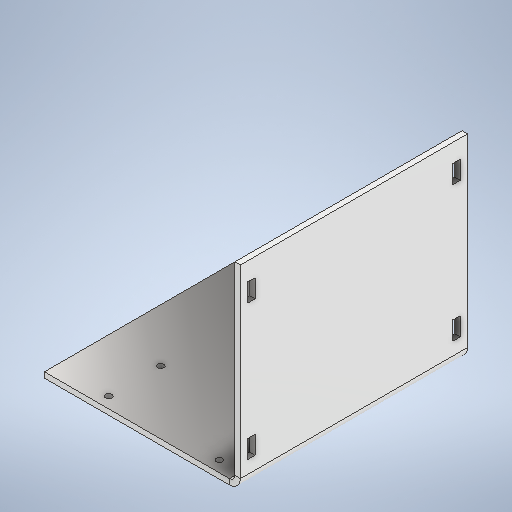
# Autodesk Inventor part: Face with CWT hole
Saved by Autodesk Inventor 2025 (Build 290162000, 162)
## iProperties
Created: 2025-08-10
Part Number: Face with CWT hole
Material: Steel, Carbon
Document SubType Name: Sheet Metal
Designer: yshis
Density: 7.85 g/cm^3
Sheet Metal Rule: Default
Appearance: Semi-Polished
Author: yshis
Autodesk Inventor part; units mm, degrees
ref_plane "YZ Plane" through (0, 0, 0) normal (1, 0, 0) x (0, 1, 0)
ref_plane "XZ Plane" through (0, 0, 0) normal (0, 1, 0) x (-1, 0, 0)
ref_plane "XY Plane" through (0, 0, 0) normal (0, 0, 1) x (1, 0, 0)
sketch "Sketch1" plane through (0, 0, 0) normal (0, 1, 0) x (-1, 0, 0)
  line L0 (0, 0) -> (107, 0)
  line L1 (107, 0) -> (107, -124)
  line L2 (107, -124) -> (0, -124)
  line L3 (0, -124) -> (0, 0)
  point P0 (53.5, -124)
  dimension "d0" = 107
  dimension "d1" = 124
  measures "d0" distance of L1.end L2.end
  measures "d1" distance of L0.end L1.end
extrude "Plate1" add sketch "Sketch1" along normal blind 3
sketch "Sketch2" plane through (-3, 0, -124) normal (1, 0, 0) x (0, 1, 0)
  line L0 (0, 124) -> (0, 0)
  line L1 (0, 0) -> (107, 0)
  line L2 (107, 0) -> (107, 124)
  line L3 (107, 124) -> (0, 124)
  constraints: 6 end point, 1 horizontal, 1 perpendicular, 1 vertical
edge flange "Flange1" height 107 angle 90 thickness 3 bend radius 3 thickness toward (1, 0, 0) relief tear relief width 3 relief depth 1.5 edges at (0, 3, -62) wall of the first edge with corners at (-3, 0, 0) (-3, 0, -124) (-3, 107, -124) (-3, 107, 0)
bend "Bend1"
corner "Corner1"
sketch "Sketch6" plane through (0, 0, 0) normal (0, -1, 0) x (1, 0, 0)
  circle A0 centre (-78, -118) radius 1.75
  line L0 (-107, -124) -> (-107, 0) projected
  line L1 (-6, -124) -> (-107, -124) projected
  circle A1 centre (-78, -34.5) radius 1.75
  circle A2 centre (-17.5, -118) radius 1.75
  circle A3 centre (-17.5, -34.5) radius 1.75
  circle A4 centre (-78, -6) radius 1.75
  line L2 (-107, 0) -> (-6, 0) projected
  circle A5 centre (-78, -89.5) radius 1.75
  circle A6 centre (-17.5, -6) radius 1.75
  circle A7 centre (-17.5, -89.5) radius 1.75
  point P0 (0, 0)
  dimension "d79" = 3.5
  dimension "d80" = 29
  dimension "d81" = 6
  dimension "d84" = 83.5
  dimension "d87" = 60.5
  dimension "d113" = 3.5
  dimension "d114" = 6
  dimension "d115" = 29
  dimension "d118" = 83.5
  dimension "d121" = 60.5
  constraints: 8 centre point, 2 horizontal, 2 vertical, 12 other
  measures "d79" diameter of A0
  measures "d80" distance from line of L0 A0.centre
  measures "d81" distance from line of L1 A0.centre
  measures "d84" distance of A0.centre A1.centre
  measures "d87" distance of A0.centre A2.centre
  measures "d113" diameter of A4
  measures "d114" distance from line of L2 A4.centre
  measures "d115" distance from line of L0 A4.centre
  measures "d118" distance of A4.centre A5.centre
  measures "d121" distance of A4.centre A6.centre
extrude "Cut4" cut sketch "Sketch6" against normal blind 3
sketch "Sketch7" plane through (0, 107, 0) normal (1, 0, 0) x (0, 0, -1)
  line L0 (120, -84) -> (116, -84)
  line L1 (116, -84) -> (116, -94)
  line L2 (116, -94) -> (120, -94)
  line L3 (120, -94) -> (120, -84)
  line L4 (124, 0) -> (124, -101) projected
  line L5 (124, -107) -> (0, -107) projected
  line L6 (120, -10) -> (116, -10)
  line L7 (116, -10) -> (116, -20)
  line L8 (116, -20) -> (120, -20)
  line L9 (120, -20) -> (120, -10)
  line L10 (8, -84) -> (4, -84)
  line L11 (4, -84) -> (4, -94)
  line L12 (4, -94) -> (8, -94)
  line L13 (8, -94) -> (8, -84)
  line L14 (8, -10) -> (4, -10)
  line L15 (4, -10) -> (4, -20)
  line L16 (4, -20) -> (8, -20)
  line L17 (8, -20) -> (8, -10)
  point P0 (124, -27)
  point P1 (124, -33)
  point P2 (12, -101)
  point P3 (12, -107)
  point P4 (12, -27)
  point P5 (12, -33)
  dimension "d92" = 10
  dimension "d93" = 4
  dimension "d94" = 4
  dimension "d95" = 13
  dimension "d105" = 74
  dimension "d108" = 112
  constraints: 32 end point, 2 horizontal, 2 parallel, 1 perpendicular, 1 vertical, 30 other
  measures "d92" distance of L0.end L1.end
  measures "d93" distance of L0.start L0.end
  measures "d94" distance between parallel lines of L4 L3
  measures "d95" distance between parallel lines of L5 L2
  measures "d105" distance of L0.start L6.start
  measures "d108" distance of L0.start L10.start
extrude "Extrusion1" cut sketch "Sketch7" against normal blind 3
equation "\"d114\" = d81"
equation "\"d115\" = d80"
equation "\"d118\" = d84"
equation "\"d121\" = d87"
equation "\"d90\" = Thickness"
equation "\"d108\" = d1 - d93 - 2 * d94"
equation "\"d24\" = Thickness"
equation "\"d25\" = BendReliefWidth"
equation "\"d26\" = BendReliefDepth"
equation "\"d27\" = MinimumRemnant"
equation "\"d28\" = TransitionRadius"
equation "\"d29\" = d0"
equation "\"d31\" = BendRadius"
equation "\"d32\" = CornerReliefSize"
equation "\"d33\" = GapSize"
equation "\"d34\" = JacobiRadiusSize"
equation "\"BendRadius\" = Thickness"
equation "\"BendReliefWidth\" = Thickness"
equation "\"BendReliefDepth\" = 0.5 * Thickness"
equation "\"CornerReliefSize\" = 4 * Thickness"
equation "\"MinimumRemnant\" = 2 * Thickness"
equation "\"TransitionRadius\" = BendRadius"
equation "\"JacobiRadiusSize\" = BendRadius"
equation "\"GapSize\" = Thickness"
equation "\"Thickness\" = 3"
body "Solid1"
